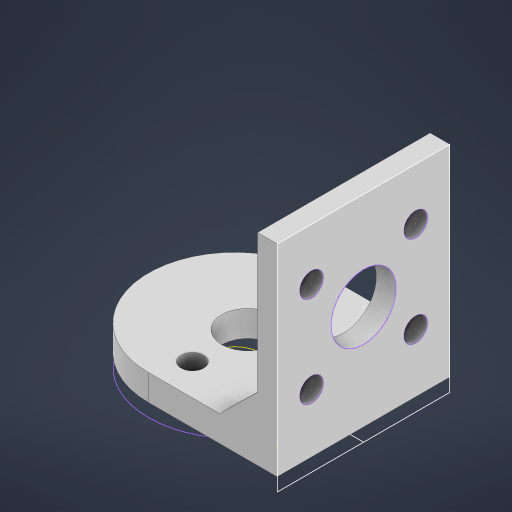
# Autodesk Inventor part: bracket bener
Saved by Autodesk Inventor 2024.3 (Build 283343000, 343)
## iProperties
Created: 2025-06-12
Part Number: bracket bener
Material: Generic
Document SubType Name: Modeling
Designer: Akbar Syihabuddin
Density: 1 g/cm^3
Appearance: Default
Author: Akbar Syihabuddin
Autodesk Inventor part; units mm, degrees
ref_plane "YZ Plane" through (0, 0, 0) normal (1, 0, 0) x (0, 1, 0)
ref_plane "XZ Plane" through (0, 0, 0) normal (0, 1, 0) x (-1, 0, 0)
ref_plane "XY Plane" through (0, 0, 0) normal (0, 0, 1) x (1, 0, 0)
sketch "Sketch1" plane through (0, 0, 0) normal (0, 1, 0) x (-1, 0, 0)
  line L0 (0, 0) -> (33, 0)
  line L1 (33, 0) -> (33, -26.5)
  line L2 (33, -26.5) -> (0, -26.5)
  line L3 (0, -26.5) -> (0, 0)
  line L4 (0, 0) -> (3, 0)
  line L5 (3, 0) -> (3, -26.5)
  line L6 (33, -13.25) -> (3, -13.25)
  circle A0 centre (19.75, -13.25) radius 4
  arc A1 (20.7334, -22.5449) -> (20.3881, -20.6583) centre (19.75, -21.75) ccw
  circle A2 centre (19.75, -21.75) radius 1.6
  circle A3 centre (19.75, -4.75) radius 1.75
  circle A4 centre (19.75, -4.75) radius 1.6
  circle A5 centre (19.75, -13.25) radius 13.25
  line L7 (19.75, -13.25) -> (33, -13.25)
  line L8 (33, -13.25) -> (19.75, -13.25)
  line L9 (33, -13.25) -> (19.75, -13.25)
  point P0 (21.6256, -13.25)
  point P1 (19.75, 0)
  point P2 (19.75, -26.5)
  dimension "d6" = 26.5
  dimension "d0" = 33
  dimension "d1" = 26.5
  dimension "d2" = 3
  dimension "d3" = 8
  dimension "d4" = 3.2
  dimension "d5" = 3.2
  dimension "d7" = 13.25
  dimension "d8" = 13.25
  constraints: 20 end point, 5 centre point, 4 coincident, 4 point on line, 2 midpoint, 2 parallel, 2 perpendicular, 2 point on circle, 1 horizontal, 3 other
  measures "d0" distance of L1.end L2.end
  measures "d1" distance of L0.end L1.end
  measures "d2" distance of L0.start L4.end
  measures "d3" diameter of A0
  measures "d4" diameter of A2
  measures "d5" diameter of A4
  measures "d7" distance of L8.start L8.end
  measures "d8" distance of L6.start L9.end
extrude "Extrusion1" add sketch "Sketch1" along normal blind 3 contours L0 A5 L6 L5 | A5 L6 A0 | L6 A5 L2 L5 | A5 L6 A0
extrude "Extrusion2" add sketch "Sketch1" along normal blind 33 contours L0 L5 L2 L3
sketch "Sketch2" plane through (0, 0, 0) normal (1, 0, 0) x (0, 0, -1)
  line L0 (0, 0) -> (0, 3) projected
  line L1 (0, 3) -> (27.1691, 3)
  line L2 (27.1691, 3) -> (27.1691, 0)
  line L3 (0, 3) -> (0, 33) projected
  line L4 (26.5, 33) -> (0, 33) projected
  line L5 (0, 3) -> (26.5, 3)
  line L6 (26.5, 3) -> (26.5, 33)
  line L7 (26.5, 33) -> (0, 33)
  line L8 (0, 33) -> (0, 3)
  line L9 (13.25, 3) -> (13.25, 33)
  line L10 (0, 18) -> (26.5, 18)
  circle A0 centre (13.25, 18) radius 5
  circle A1 centre (21.25, 11) radius 1.8
  circle A2 centre (21.25, 11) radius 1.8
  circle A3 centre (21.25, 25) radius 1.8
  circle A4 centre (21.25, 25) radius 1.8
  circle A5 centre (5.25, 25) radius 1.8
  circle A6 centre (5.25, 25) radius 1.8
  circle A7 centre (5.25, 11) radius 1.8
  circle A8 centre (5.25, 11) radius 1.8
  point P0 (13.25, 18)
  constraints: 16 end point, 9 centre point, 5 midpoint, 4 coincident, 2 horizontal, 2 parallel, 2 perpendicular
extrude "Extrusion3" cut sketch "Sketch2" against normal blind 33 contours A0 L10 L9 | L9 L10 A0 | A0 L9 L10 | L9 A0 L10 | A1 | A3 | A5 | A7
sketch "Sketch3" plane through (0, 0, 0) normal (1, 0, 0) x (0, 0, -1)
  line L0 (26.5, 3) -> (26.5, 33) projected
  line L1 (0, 0) -> (26.5, 0)
  line L2 (26.5, 0) -> (26.5, 33)
  line L3 (26.5, 33) -> (0, 33)
  line L4 (0, 33) -> (0, 0)
  circle A0 centre (5.25, 11) radius 1.8 projected
  circle A1 centre (5.25, 11) radius 1.8
  circle A2 centre (13.25, 18) radius 5 projected
  circle A3 centre (13.25, 18) radius 5
  circle A4 centre (5.25, 25) radius 1.8 projected
  circle A5 centre (5.25, 25) radius 1.8
  circle A6 centre (21.25, 25) radius 1.8 projected
  circle A7 centre (21.25, 25) radius 1.8
  circle A8 centre (21.25, 11) radius 1.8 projected
  circle A9 centre (21.25, 11) radius 1.8
  constraints: 8 end point, 5 centre point, 5 coincident, 2 parallel, 1 horizontal, 1 perpendicular
sketch "Sketch4" plane through (0, 0, 0) normal (0, -1, 0) x (1, 0, 0)
  circle A0 centre (-19.75, -13.25) radius 4 projected
  circle A1 centre (-19.75, -13.25) radius 13.25
  line L0 (0, 0) -> (0, -26.5) projected
  line L1 (0, -13.25) -> (-6.5, -13.25)
  constraints: 2 end point, 1 coincident, 1 horizontal alignment, 1 midpoint, 1 perpendicular, 2 other
sketch "Sketch5" plane through (0, 3, 0) normal (0, 1, 0) x (1, 0, 0)
  line L0 (-4.5842, 26.562) -> (-4.5842, 0.062)
  arc A0 (-16.8508, 4.0171) -> (-17.1961, 5.9037) centre (-17.8342, 4.812) ccw
  line L1 (-4.5842, 13.312) -> (-17.8342, 13.312)
  line L2 (-17.8342, 13.312) -> (-4.5842, 13.312)
  circle A1 centre (-17.8342, 4.812) radius 1.6
  circle A2 centre (-17.8342, 13.312) radius 4
  circle A3 centre (-17.8342, 21.812) radius 1.6
  circle A4 centre (-17.8342, 21.812) radius 1.75
  circle A5 centre (-17.8342, 13.312) radius 13.25
  line L3 (-4.5842, 13.312) -> (-17.8342, 13.312)
  circle A6 centre (-19.75, 4.75) radius 1.75 projected
  circle A7 centre (-19.75, 4.75) radius 1.75
  circle A8 centre (-19.75, 13.25) radius 4 projected
  circle A9 centre (-19.75, 13.25) radius 4
  circle A10 centre (-19.75, 21.75) radius 1.6 projected
  circle A11 centre (-19.75, 21.75) radius 1.6
  point P0 (0, 0)
  point P1 (-15.9586, 13.312)
  point P2 (-18.6665, 9.3996)
  point P3 (-18.9177, 17.1625)
  point P4 (-18.8788, 20.408)
  point P5 (-18.9674, 23.1455)
  point P6 (-18.6168, 3.4165)
  point P7 (-18.7054, 6.154)
  point P8 (-18.8335, 23.0615)
  point P9 (-18.7506, 20.5005)
  dimension "d19" = 26.5
  dimension "d15" = 26.5
  dimension "d16" = 8
  dimension "d17" = 3.2
  dimension "d18" = 3.2
  dimension "d20" = 13.25
  dimension "d21" = 13.25
  constraints: 8 centre point, 8 end point, 7 coincident, 2 point on circle, 1 horizontal alignment, 1 midpoint, 2 other
  measures "d15" distance of L0.start L0.end
  measures "d16" diameter of A2
  measures "d17" diameter of A1
  measures "d18" diameter of A3
  measures "d20" distance of L1.start L1.end
  measures "d21" distance of L3.start L3.end
extrude "Extrusion4" add sketch "Sketch5" against normal blind 3 contours A2 A8 | A1 A6 | A4 A10 picked at (-23.0854, 13.3028) picked at (-20.7824, 4.5119)
extrude "Extrusion5" cut sketch "Sketch5" against normal blind 3 contours A2 A8 L1 | L1 A8 A2 | A1 A6 | A3 A10 | A3 A10 A4 | A10 A3 picked at (-17.4422, 5.0312) picked at (-17.5062, 23.4206)
sketch "Sketch6" plane through (0, 3, 0) normal (0, 1, 0) x (1, 0, 0)
  circle A0 centre (-17.8342, 13.312) radius 4 projected
  circle A1 centre (-17.8342, 13.312) radius 4
  circle A2 centre (-17.8342, 21.812) radius 1.75 projected
  circle A3 centre (-17.8342, 21.812) radius 1.75
  circle A4 centre (-17.8342, 4.812) radius 1.6 projected
  circle A5 centre (-17.8342, 4.812) radius 1.75
  arc A6 (-19.75, 26.5) -> (-19.75, 0) centre (-19.75, 13.25) ccw projected
  circle A7 centre (-19.75, 13.25) radius 13.25
  line L0 (-3, 0) -> (-3, 26.5) projected
  line L1 (-19.75, 0) -> (-3, 0)
  line L2 (-3, 0) -> (-3, 26.5)
  line L3 (-3, 26.5) -> (-19.75, 26.5)
  point P0 (0, 0)
  dimension "d26" = 3.5
  constraints: 6 end point, 4 centre point, 4 coincident, 2 perpendicular, 1 collinear, 1 tangent
  measures "d26" diameter of A5
extrude "Extrusion6" add sketch "Sketch6" along normal blind 3 contours A7 A6 | L3 L0 L1 A7
sketch "Sketch7" plane through (0, 0, 0) normal (0, -1, 0) x (1, 0, 0)
  line L0 (0, -26.5) -> (-34.8144, -26.5)
  line L1 (-34.8144, -26.5) -> (-34.8144, 0)
  line L2 (-34.8144, 0) -> (0, 0)
  line L3 (0, 0) -> (0, -26.5)
  constraints: 8 end point, 2 parallel, 1 horizontal, 1 perpendicular
extrude "Extrusion7" cut sketch "Sketch7" against normal blind 2
sketch "Sketch8" plane through (0, 33, -26.5) normal (0, 0, -1) x (-1, 0, 0)
  line L0 (3, -27) -> (3, 0) projected
  line L1 (3, -21.2559) -> (8.8185, -27)
  line L2 (3, -27) -> (19.75, -27) projected
  line L3 (3, -21.2559) -> (3, -27)
  line L4 (3, -27) -> (8.8185, -27)
  point P0 (0, -33)
  constraints: 6 end point, 2 point on line, 1 collinear, 1 vertical
extrude "Extrusion8" add sketch "Sketch8" against normal blind 2
sketch "Sketch9" plane through (-3, 33, 0) normal (0, 0, 1) x (1, 0, 0)
  line L0 (0, -21.2559) -> (-5.8185, -27) projected
  line L1 (-5.8185, -27) -> (0, -21.2559)
  line L2 (0, -27) -> (0, 0) projected
  line L3 (0, -21.2559) -> (0, -27)
  line L4 (0, -27) -> (-5.8185, -27)
  point P0 (3, -33)
  constraints: 6 end point, 1 collinear, 1 perpendicular
extrude "Extrusion9" add sketch "Sketch9" against normal blind 2
sketch "Sketch10" plane through (0, 6, 0) normal (0, 1, 0) x (1, 0, 0)
  point P0 (0, 0)
body "Solid1"
